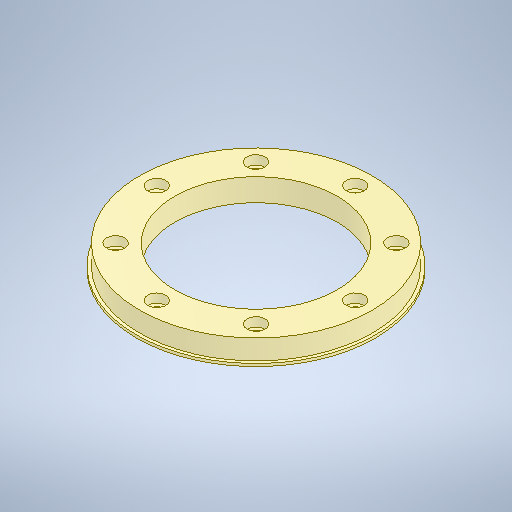
# Autodesk Inventor part: DMF 01 31 Барабан Опорное кольцо НОС v2.1
Saved by Autodesk Inventor 2026.2 (Build 302298000, 298)
## iProperties
Created: 2024-04-28
Part Number: DMF 01 31 Барабан Опорное кольцо НОС v2.1
Material: Generic
Document SubType Name: Sheet Metal
Designer: pokla
Density: 1 g/cm^3
Appearance: Nylon 6
Stock Number: Опорное_Кольцо_Нос
Sheet Metal Rule: Default
Author: pokla
Autodesk Inventor part; units mm, degrees
ref_plane "YZ Plane" through (0, 0, 0) normal (1, 0, 0) x (0, 1, 0)
ref_plane "XZ Plane" through (0, 0, 0) normal (0, 1, 0) x (-1, 0, 0)
ref_plane "XY Plane" through (0, 0, 0) normal (0, 0, 1) x (1, 0, 0)
sketch "Sketch6" plane through (0, 0, 0) normal (0, 0, 1) x (1, 0, 0)
  line L0 (90, 0) -> (90, 25)
  line L1 (90, 25) -> (129, 25)
  line L2 (129, 25) -> (129, 3)
  line L3 (129, 3) -> (132.5, 3)
  line L4 (132.5, 3) -> (132.5, 0)
  line L5 (132.5, 0) -> (90, 0)
  line L6 (0, 0) -> (0, 25)
  point P0 (0, 0)
  dimension "d27" = 180
  dimension "d28" = 258
  dimension "d29" = 265
  dimension "d30" = 3
  dimension "d31" = 25
  constraints: 14 end point, 6 perpendicular, 2 point on line, 1 coincident, 1 vertical
  measures "d27" diameter of L0 L6
  measures "d28" diameter of L2 L6
  measures "d29" diameter of L4 L6
  measures "d30" distance between parallel lines of L5 L3
  measures "d31" distance between parallel lines of L5 L1
revolve "Revolution1" add sketch "Sketch6" angle 360 about axis through (0, 0, 0) along (0, 1, 0)
sketch "Sketch7" plane through (0, 25, 0) normal (0, 1, 0) x (1, 0, 0)
  circle A0 centre (0, 0) radius 110
  point P0 (0, 110)
  dimension "d33" = 220
  constraints: 2 vertical alignment, 1 coincident, 2 other
hole "Hole2" at (0, 25, -110) direction (0, -1, 0) diameter 11 end through all counterbore diameter 20 counterbore depth 10
pattern_circular "Circular Pattern3" count 8 over 360 about axis through (0, -10, 0) along (0, 1, 0) of "Hole2"
equation "\"d39\" = Thickness"
equation "\"Thickness\" = 40"
body "Solid2"
